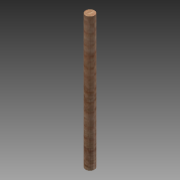
# Autodesk Inventor part: 轴
Saved by Autodesk Inventor 2013 (Build 170138000, 138)
## iProperties
Created: 2012-10-03
Part Number: 轴
Material: 木材(桦木)
Document SubType Name: Modeling
Designer: Zhensheng
Density: 0.55 g/cm^3
Mass: 6.47953 g
Surface Area: 48.6947 cm^2
Volume: 11.781 cm^3
Author: Zhensheng
Autodesk Inventor part; units mm, degrees
ref_plane "YZ Plane" through (0, 0, 0) normal (1, 0, 0) x (0, 1, 0)
ref_plane "XZ Plane" through (0, 0, 0) normal (0, 1, 0) x (-1, 0, 0)
ref_plane "XY Plane" through (0, 0, 0) normal (0, 0, 1) x (1, 0, 0)
sketch "草图1" plane through (0, 0, 0) normal (0, 0, 1) x (1, 0, 0)
  circle A0 centre (0, 0) radius 5
  dimension "轴径" = 10
  constraints: 1 centre point, 1 coincident
  measures "轴径" diameter of A0
extrude "拉伸1" add sketch "草图1" along normal blind 150
